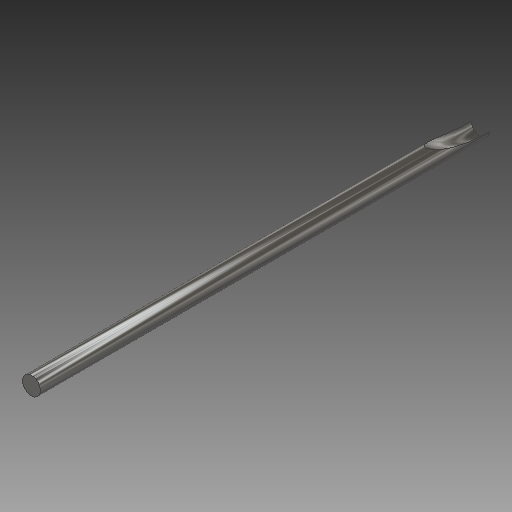
# Autodesk Inventor part: バネねじり270.z3.2
Saved by Autodesk Inventor 2020 (Build 240168000, 168)
## iProperties
Created: 2018-12-29
Part Number: バネねじり270.z3.2
Material: 鋼、高強度、低合金
Document SubType Name: Modeling
Designer: 雪村
Density: 7.85 g/cm^3
Appearance: 鋼 - つや出し
Mass: 0.246079 g
Surface Area: 1.14471 cm^2
Volume: 0.0313477 cm^3
Author: 雪村
Autodesk Inventor part; units mm, degrees
ref_plane "YZ Plane" through (0, 0, 0) normal (1, 0, 0) x (0, 1, 0)
ref_plane "XY Plane" through (0, 0, 0) normal (0, 0, 1) x (1, 0, 0)
sketch "スケッチ1" plane through (0, 0, 0) normal (0, 0, 1) x (1, 0, 0)
  circle A0 centre (0, 0) radius 0.6
  dimension "d0" = 1.2
  constraints: 1 centre point, 1 coincident
  measures "d0" diameter of A0
extrude "押し出し1" add sketch "スケッチ1" along normal blind 30
ref_plane "作業平面1" through (0, 5.6, 0) normal (0, 1, 0) x (-1, 0, 0)
sketch "スケッチ3" plane through (0, 5.6, 0) normal (0, 1, 0) x (-1, 0, 0)
  circle A0 centre (0, -5.6) radius 0.6
  line L0 (0, -5) -> (2.6208, -5) construction
  line L1 (0, 0) -> (5.2204, 0)
  dimension "d6" = 1.2
  dimension "d7" = 5
  constraints: 4 end point, 3 horizontal, 2 vertical alignment, 2 other
  measures "d7" distance from line of L0 L1.start
revolve "回転1" cut sketch "スケッチ3" angle 360 about axis through (0, 5.6, 0) along (-1, 0, 0)
